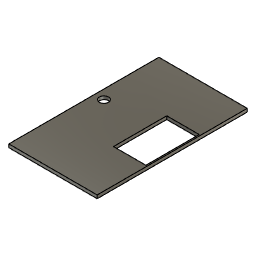
zavirani2 (Autodesk Fusion 360 design; units mm, degrees)
Autodesk Fusion 360 part; units mm, degrees
sketch "Sketch1" plane through (0, 0, 0) normal (0, 0, 1) x (1, 0, 0)
  line L0 (0, 0) -> (38.2, 0)
  line L1 (38.2, 0) -> (38.2, 66.3)
  line L2 (38.2, 66.3) -> (0, 66.3)
  line L3 (0, 66.3) -> (0, 0)
  dimension "d1" = 38.2
  dimension "d2" = 66.3
  constraint horizontal L0
  constraint vertical L1
  constraint horizontal L2
  constraint vertical L3
  constraint coincident L0.start L3.end
  measures "d1" distance of L0.start L0.end
  measures "d2" distance of L0.start L2.end
extrude "Extrude1" add sketch "Sketch1" along normal blind 1.3
sketch "Sketch2" plane through (0, 0, 1.3) normal (0, 0, 1) x (-1, 0, 0)
  line L0 (0, -66.3) -> (0, 0)
  line L1 (0, 0) -> (-38.2, 0)
  line L2 (-38.2, 0) -> (-38.2, -66.3)
  line L3 (-38.2, -66.3) -> (0, -66.3)
  line L4 (-0.6, -63.65) -> (-37.6, -63.65)
  line L5 (-37.6, -63.65) -> (-37.6, -2.65)
  line L6 (-37.6, -2.65) -> (-0.6, -2.65)
  line L7 (-0.6, -2.65) -> (-0.6, -63.65)
  line L8 (-37.6, -21.65) -> (-23.6, -21.65)
  line L9 (-23.6, -21.65) -> (-23.6, -44.65)
  line L10 (-23.6, -44.65) -> (-37.6, -44.65)
  line L11 (-37.6, -44.65) -> (-37.6, -21.65)
  line L12 (-0.6, -37.15) -> (-4, -37.15) construction
  circle A0 centre (-4, -37.15) radius 1.5
  dimension "d5" = 37
  dimension "d6" = 61
  dimension "d7" = 2.65
  dimension "d8" = 0.6
  dimension "d9" = 14
  dimension "d10" = 19
  dimension "d11" = 19
  dimension "d12" = 26.5
  dimension "d13" = 3
  constraint horizontal L4
  constraint vertical L5
  constraint horizontal L6
  constraint vertical L7
  constraint horizontal L8
  constraint vertical L9
  constraint horizontal L10
  constraint vertical L11
  constraint coincident L5 L8.start
  constraint coincident L7 L12.start
  constraint perpendicular L7 L12
  constraint coincident L12.end A0.centre
  measures "d5" distance of L4.start L4.end
  measures "d6" distance of L4.start L6.end
  measures "d7" distance of L3 L4
  measures "d8" distance of L0 L7
  measures "d9" distance of L8.start L8.end
  measures "d10" distance of L6 L8
  measures "d11" distance of L4 L10
  measures "d12" distance of L4 L12
  measures "d13" diameter of A0
extrude "Extrude2" cut sketch "Sketch2" against normal blind 78 contours A0
extrude "Extrude3" cut sketch "Sketch2" against normal blind 2 contours L5 L8 L9 L10 L11
extrude "Extrude4" cut 1 faces at (25.4667, 66.3, 0.4333) along direction (0, -1, 0) blind 0.95
extrude "Extrude5" add 1 faces at (20.6, 7.2167, 1.3) along direction (0, 0, 1) blind 0.1
extrude "Extrude6" cut 1 faces at (25.4667, 65.35, 0.4667) along direction (0, -1, 0) blind 0.5
sketch "Sketch3" plane through (0, 0, 1.4) normal (0, 0, 1) x (-1, 0, 0)
  line L0 (-23.6, -21.65) -> (-23.6, -44.65)
  line L1 (-23.6, -44.65) -> (-37.6, -44.65)
  line L2 (-37.6, -44.65) -> (-37.6, -21.65)
  line L3 (-37.6, -21.65) -> (-23.6, -21.65)
  circle A0 centre (-4, -37.15) radius 1.5
  line L4 (-38.2, -64.85) -> (0, -64.85)
  line L5 (0, -64.85) -> (0, 0)
  line L6 (0, 0) -> (-38.2, 0)
  line L7 (-38.2, 0) -> (-38.2, -64.85)
  circle A1 centre (-4, -37.15) radius 2
  dimension "d24" = 4
  constraint concentric A0 A1
  measures "d24" diameter of A1
extrude "Extrude7" cut sketch "Sketch3" against normal blind 4 contours A1
equation "d18 = -2.65 mm + 1.7 mm"
